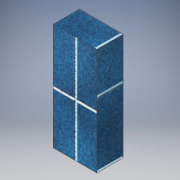
# Autodesk Inventor part: battery
Saved by Autodesk Inventor 2017 (Build 210142000, 142)
## iProperties
Created: 2016-11-05
Part Number: battery
Material: Generic
Document SubType Name: Modeling
Designer: radrajith
Density: 1 g/cm^3
Appearance: Default
Author: radrajith
Autodesk Inventor part; units mm, degrees
ref_plane "YZ Plane" through (0, 0, 0) normal (1, 0, 0) x (0, 1, 0)
ref_plane "XZ Plane" through (0, 0, 0) normal (0, 1, 0) x (-1, 0, 0)
ref_plane "XY Plane" through (0, 0, 0) normal (0, 0, 1) x (1, 0, 0)
sketch "Sketch3" plane through (0, 0, 0) normal (0, 0, 1) x (1, 0, 0)
  line L0 (0, 0) -> (25.6, 0)
  line L1 (25.6, 0) -> (25.6, 63)
  line L2 (25.6, 63) -> (0, 63)
  line L3 (0, 63) -> (0, 0)
  dimension "d0" = 25.6
  dimension "d1" = 63
  constraints: 8 end point, 2 parallel, 1 horizontal, 1 perpendicular
  measures "d0" distance of L2.end L1.end
  measures "d1" distance of L1.end L0.end
extrude "Extrusion1" add sketch "Sketch3" along normal blind 15.5
sketch "Sketch4" plane through (0, 0, 0) normal (0, 0, -1) x (-1, 0, 0)
  line L0 (-16.1, 56.5) -> (-9.5, 56.5)
  line L1 (-9.5, 56.5) -> (-9.5, 53)
  line L2 (-9.5, 53) -> (-16.1, 53)
  line L3 (-16.1, 53) -> (-16.1, 56.5)
  line L4 (-25.6, 0) -> (-25.6, 63) projected
  line L5 (0, 63) -> (0, 0) projected
  dimension "d4" = 9.5
  dimension "d5" = 9.5
  constraints: 8 end point, 2 parallel, 1 horizontal, 1 perpendicular
  measures "d4" distance between parallel lines of L4 L3
  measures "d5" distance between parallel lines of L5 L1
extrude "Extrusion2" add sketch "Sketch4" along normal blind 2
body "Solid1"
